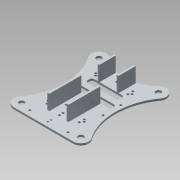
# Autodesk Inventor part: basebawahV2
Saved by Autodesk Inventor 2015 SP1 (Build 190203100, 203)
## iProperties
Created: 2015-01-14
Part Number: basebawahV2
Material: ABS Plastic
Document SubType Name: Modeling
Designer: Rafi Kurnia Putra
Density: 1.06 g/cm^3
Appearance: Default
Mass: 42.2508 g
Surface Area: 270.463 cm^2
Volume: 39.8593 cm^3
Author: Rafi Kurnia Putra
Autodesk Inventor part; units mm, degrees
ref_plane "YZ Plane" through (0, 0, 0) normal (1, 0, 0) x (0, 1, 0)
ref_plane "XZ Plane" through (0, 0, 0) normal (0, 1, 0) x (-1, 0, 0)
ref_plane "XY Plane" through (0, 0, 0) normal (0, 0, 1) x (1, 0, 0)
sketch "Sketch1" plane through (0, 0, 0) normal (0, 1, 0) x (-1, 0, 0)
  circle A0 centre (46.65, 60.8866) radius 4.25
  circle A1 centre (25.375, 42.175) radius 1.75
  circle A2 centre (28.625, 37.55) radius 1.75
  circle A3 centre (46.65, -60.8866) radius 4.25
  circle A4 centre (25.375, -42.175) radius 1.75
  circle A5 centre (28.625, -37.55) radius 1.75
  circle A6 centre (25.5, -34.24) radius 1.75
  circle A7 centre (25.5, 34.24) radius 1.75
  arc A8 (55.3297, 52.2069) -> (37.9702, 69.5664) centre (46.65, 60.8866) ccw
  arc A9 (37.9702, -69.5664) -> (55.3297, -52.2069) centre (46.65, -60.8866) ccw
  circle A10 centre (35.7091, 28.8987) radius 1.75
  circle A11 centre (38.6257, 37.55) radius 1.75
  circle A12 centre (28.8757, 53.55) radius 1.75
  line L0 (12.2659, 71.7451) -> (15.3224, 61.7249)
  arc A13 (22.1689, 58.6296) -> (37.9702, 69.5664) centre (0.0022, 107.5388) ccw
  arc A14 (15.3224, 61.7249) -> (22.1689, 58.6296) centre (20.1049, 63.1837) ccw
  circle A15 centre (-25.375, 42.175) radius 1.75
  circle A16 centre (-28.625, 37.55) radius 1.75
  circle A17 centre (-46.65, 60.8866) radius 4.25
  circle A18 centre (-25.375, -42.175) radius 1.75
  circle A19 centre (-28.625, -37.55) radius 1.75
  circle A20 centre (-46.65, -60.8866) radius 4.25
  circle A21 centre (-25.5, -34.24) radius 1.75
  circle A22 centre (-25.5, 34.24) radius 1.75
  arc A23 (-37.9702, 69.5664) -> (-55.3297, 52.2069) centre (-46.65, 60.8866) ccw
  arc A24 (-55.3297, -52.2069) -> (-37.9702, -69.5664) centre (-46.65, -60.8866) ccw
  circle A25 centre (-28.8757, 53.55) radius 1.75
  circle A26 centre (-38.6257, 37.55) radius 1.75
  circle A27 centre (-35.7091, 28.8987) radius 1.75
  line L1 (-12.2659, 71.7451) -> (-15.3224, 61.7249)
  arc A28 (-37.9702, 69.5664) -> (-22.1689, 58.6296) centre (-0.0022, 107.5388) ccw
  arc A29 (-22.1689, 58.6296) -> (-15.3224, 61.7249) centre (-20.1049, 63.1837) ccw
  circle A30 centre (0, 42.1912) radius 1.75
  arc A31 (37.9702, -69.5664) -> (-37.9702, -69.5664) centre (0, -107.5245) ccw
  line L2 (10.3529, 73.1616) -> (-10.3529, 73.1616)
  arc A32 (-55.3297, -52.2069) -> (-55.3297, 52.2069) centre (-134.1138, 0) ccw
  arc A33 (55.3297, 52.2069) -> (55.3297, -52.2069) centre (134.1138, 0) ccw
  arc A34 (12.2659, 71.7451) -> (10.3529, 73.1616) centre (10.3529, 71.1616) ccw
  arc A35 (-10.3529, 73.1616) -> (-12.2659, 71.7451) centre (-10.3529, 71.1616) ccw
  arc A36 (25.375, -21.8592) -> (21.875, -18.3592) centre (21.875, -21.8592) ccw
  arc A37 (21.875, -28.3427) -> (25.375, -24.8427) centre (21.875, -24.8427) ccw
  arc A38 (-25.375, -24.8427) -> (-21.875, -28.3427) centre (-21.875, -24.8427) ccw
  arc A39 (-21.875, -18.3592) -> (-25.375, -21.8592) centre (-21.875, -21.8592) ccw
  line L3 (-21.875, -18.3592) -> (21.875, -18.3592)
  line L4 (21.875, -28.3427) -> (-21.875, -28.3427)
  line L5 (-25.375, -21.8592) -> (-25.375, -24.8427)
  line L6 (25.375, -21.8592) -> (25.375, -24.8427)
  circle A40 centre (0, 61.1616) radius 1.25
  circle A41 centre (0, 66.1616) radius 1.25
  circle A42 centre (0, -42.1912) radius 1.75
  circle A43 centre (0, -48.0131) radius 1.75
  circle A44 centre (0, 48.0131) radius 1.75
  circle A45 centre (-34.6272, 13.8987) radius 1.75
  circle A46 centre (-34.6272, -13.8987) radius 1.75
  circle A47 centre (34.6272, 13.8987) radius 1.75
  circle A48 centre (34.6272, -13.8987) radius 1.75
  point P0 (57.609, 54.4281)
  point P1 (16.8957, 56.5674)
  point P2 (-0.0035, -53.835)
  point P3 (-57.609, 54.4281)
  point P4 (-16.8957, 56.5674)
  point P5 (0.0035, -53.835)
  point P6 (39.6019, 0)
  point P7 (-39.6019, 0)
  point P8 (25.25, -18.3592)
  point P9 (0, -18.3592)
  point P10 (-25.25, -18.3592)
  point P11 (46.65, -73.1616)
  point P12 (0, -73.1616)
  point P13 (46.65, 73.1616)
  point P14 (46.65, -73.1616)
  point P15 (-40.6295, 13.8987)
  dimension "d105" = 3.5
  dimension "d106" = 3.5
  dimension "d198" = 16
  dimension "d199" = 8.6513
  dimension "d244" = 5
  dimension "d247" = 79.2039
  dimension "d248" = 2
  dimension "d249" = 3.5
  dimension "d250" = 2.5
  dimension "d251" = 2.5
  dimension "d252" = 146.3233
  dimension "d253" = 146.3233
  dimension "d258" = 6.0022
  dimension "d259" = 27.7974
  dimension "d260" = 69.2545
  dimension "d263" = 5.8219
  dimension "d264" = 5.8219
  dimension "d265" = 5.8219
  dimension "d266" = 46.9879
  dimension "d267" = 12.0227
  dimension "d271" = 46.9879
  dimension "d272" = 12.0227
  constraints: 49 centre point, 42 point on circle, 14 end point, 6 tangent, 3 coincident, 2 equal radius, 2 point on line, 1 horizontal, 1 parallel, 1 perpendicular, 2 other
  measures "d105" diameter of A6
  measures "d106" diameter of A7
  measures "d198" vertical distance of A12.centre A11.centre
  measures "d199" vertical distance of A10.centre A11.centre
  measures "d244" radius of A14
  measures "d247" distance of point (-39.602, 0) point (39.602, 0)
  measures "d248" radius of A34
  measures "d249" radius of A36
  measures "d250" diameter of A40
  measures "d251" diameter of A41
  measures "d252" distance from line of L2 point (0, -73.162)
  measures "d253" distance of point (46.65, -73.162) point (46.65, 73.162)
  measures "d258" distance of A45.centre point (-40.629, 13.899)
  measures "d259" distance of A46.centre A45.centre
  measures "d260" distance of A47.centre A45.centre
  measures "d263" distance of A43.centre point (-0.004, -53.835)
  measures "d264" distance of A42.centre A43.centre
  measures "d265" distance of A30.centre A44.centre
  measures "d266" vertical distance of A45.centre A17.centre
  measures "d267" horizontal distance of A45.centre A17.centre
  measures "d271" vertical distance of A46.centre A20.centre
  measures "d272" horizontal distance of A46.centre A20.centre
extrude "Extrusion14" add sketch "Sketch1" along normal mid plane 3
sketch "Sketch14" plane through (0, -1.5, 0) normal (0, -1, 0) x (1, 0, 0)
  line L0 (31.815, 0) -> (31.815, -5.9519)
  arc A0 (28.315, -9.4519) -> (31.815, -5.9519) centre (28.315, -5.9519) ccw
  arc A1 (28.315, -9.4519) -> (28.625, -9.4382) centre (28.315, -5.9519) ccw
  line L1 (28.315, -9.4519) -> (0.0544, -9.4519)
  line L2 (28.315, 9.4519) -> (0.0544, 9.4519)
  arc A2 (31.815, 5.9519) -> (28.315, 9.4519) centre (28.315, 5.9519) ccw
  line L3 (31.815, 0) -> (31.815, 5.9519)
  arc A3 (28.625, 9.4382) -> (28.315, 9.4519) centre (28.315, 5.9519) ccw
  line L4 (-28.315, -9.4519) -> (-0.0544, -9.4519)
  line L5 (-31.815, 0) -> (-31.815, -5.9519)
  arc A4 (-31.815, -5.9519) -> (-28.315, -9.4519) centre (-28.315, -5.9519) ccw
  arc A5 (-28.625, -9.4382) -> (-28.315, -9.4519) centre (-28.315, -5.9519) ccw
  line L6 (-28.315, 9.4382) -> (-0.0544, 9.445)
  arc A6 (-28.315, 9.4382) -> (-28.6259, 9.4244) centre (-28.315, 5.9382) ccw
  arc A7 (-28.315, 9.4382) -> (-31.815, 5.9519) centre (-28.315, 5.9382) ccw
  line L7 (-31.815, 0) -> (-31.815, 5.9519)
  line L8 (-28.315, 9.4382) -> (28.625, 9.4382)
  line L9 (28.625, -9.4382) -> (-28.625, -9.4382)
  line L10 (-31.815, 5.9519) -> (-31.815, -5.9519)
  line L11 (31.815, 5.9519) -> (31.815, -5.9519)
  point P0 (0, 0)
  point P1 (0, 0)
  dimension "d268" = 63.63
  constraints: 24 end point, 20 point on circle, 8 centre point, 2 collinear, 2 parallel
  measures "d268" distance of L5.start L0.start
extrude "Extrusion15" cut sketch "Sketch14" against normal blind 3
sketch "Sketch15" plane through (0, 1.5, 0) normal (0, 1, 0) x (1, 0, 0)
  arc A0 (-46.65, -73.1616) -> (-37.9702, -69.5664) centre (-46.65, -60.8866) ccw
  arc A1 (-22.1689, -58.6296) -> (-37.9702, -69.5664) centre (-0.0022, -107.5388) ccw
  arc A2 (-15.3224, -61.7249) -> (-22.1689, -58.6296) centre (-20.1049, -63.1837) ccw
  line L0 (-15.3224, -61.7249) -> (-12.2659, -71.7451)
  arc A3 (-12.2659, -71.7451) -> (-10.3529, -73.1616) centre (-10.3529, -71.1616) ccw
  arc A4 (10.3529, -73.1616) -> (12.2659, -71.7451) centre (10.3529, -71.1616) ccw
  line L1 (12.2659, -71.7451) -> (15.3224, -61.7249)
  arc A5 (22.1689, -58.6296) -> (15.3224, -61.7249) centre (20.1049, -63.1837) ccw
  arc A6 (37.9702, -69.5664) -> (22.1689, -58.6296) centre (0.0022, -107.5388) ccw
  arc A7 (37.9702, -69.5664) -> (46.65, -73.1616) centre (46.65, -60.8866) ccw
  arc A8 (-46.65, -73.1616) -> (-37.9702, -69.5664) centre (-46.65, -60.8866) ccw
  line L2 (-46.65, -73.1616) -> (-10.3529, -73.1616)
  line L3 (10.3529, -73.1616) -> (46.65, -73.1616)
  line L4 (31.815, -5.9519) -> (31.815, 3.5)
  arc A9 (28.625, -9.4382) -> (31.815, -5.9519) centre (28.315, -5.9519) ccw
  line L5 (-28.315, -9.4382) -> (28.625, -9.4382)
  arc A10 (-31.815, -5.9519) -> (-28.315, -9.4382) centre (-28.315, -5.9382) ccw
  line L6 (-31.815, 3.5) -> (-31.815, -5.9519)
  line L7 (28.315, 0) -> (-28.315, 0)
  arc A11 (28.315, 0) -> (31.815, 3.5) centre (28.315, 3.5) ccw
  arc A12 (-31.815, 3.5) -> (-28.315, 0) centre (-28.315, 3.5) ccw
  dimension "d278" = 3.5
  dimension "d279" = 3.5
  constraints: 26 point on circle, 21 centre point, 16 end point, 4 tangent, 2 horizontal
  measures "d278" radius of A11
  measures "d279" radius of A12
extrude "Extrusion16" add sketch "Sketch15" against normal blind 3 contours A0 A1 A2 L0 A3 L2 | A4 L1 A5 A6 A7 L3
extrude "Extrusion17" add sketch "Sketch15" against normal blind 3 contours A9 L5 A10 L6 A12 L7 A11 L4
sketch "Sketch18" plane through (0, -1.5, 0) normal (0, -1, 0) x (1, 0, 0)
  arc A0 (23.8353, 3.8182) -> (25.559, 5.5419) centre (22.3772, 7) ccw projected
  line L0 (25.8772, 15.6487) -> (25.8772, 7) projected
  line L1 (22.3772, 3.5) -> (-22.3773, 3.5) projected
  circle A1 centre (20.8772, 8.5) radius 1.75
  circle A2 centre (-20.8772, 8.5) radius 1.75
  point P0 (0, 0)
  dimension "d285" = 5
  dimension "d286" = 5
  constraints: 2 centre point
  measures "d285" distance from line of A1.centre L1
  measures "d286" distance from line of A1.centre L0
extrude "Extrusion18" cut sketch "Sketch18" against normal up to next
sketch "Sketch19" plane through (0, -1.5, 0) normal (0, -1, 0) x (1, 0, 0)
  circle A0 centre (-30, 64.6618) radius 1.75
  line L0 (0, 0) -> (0, 78.7482)
  line L1 (-36.7454, 69.6618) -> (36.7451, 69.6619)
  circle A1 centre (-9, 28.5) radius 1.75
  line L2 (22.3772, 3.5) -> (-22.3773, 3.5)
  circle A2 centre (30, 64.6618) radius 1.75
  circle A3 centre (9, 28.5) radius 1.75
  dimension "d289" = 3.5
  dimension "d300" = 30
  dimension "d301" = 5
  dimension "d302" = 3.5
  dimension "d303" = 25
  dimension "d304" = 9
  constraints: 6 end point, 4 centre point, 2 symmetric about line, 1 vertical, 8 other
  measures "d289" diameter of A0
  measures "d300" distance from line of A0.centre L0
  measures "d301" distance from line of A0.centre L1
  measures "d302" diameter of A1
  measures "d303" distance from line of A1.centre L2
  measures "d304" distance from line of L0 A1.centre
sketch "Sketch20" plane through (0, -1.5, 0) normal (0, -1, 0) x (1, 0, 0)
  circle A0 centre (-35.7091, 28.8987) radius 1.75 projected
  circle A1 centre (-20.8772, 8.5) radius 1.75 projected
  circle A2 centre (20.8772, 8.5) radius 1.75 projected
  circle A3 centre (35.7091, 28.8987) radius 1.75 projected
  circle A4 centre (-38.6257, 37.55) radius 1.75 projected
  circle A5 centre (38.6257, 37.55) radius 1.75 projected
  circle A6 centre (-28.8757, 53.55) radius 1.75 projected
  circle A7 centre (28.8757, 53.55) radius 1.75 projected
  point P0 (0, 0)
extrude "Extrusion19" add sketch "Sketch20" against normal blind 3
extrude "Extrusion20" cut sketch "Sketch19" against normal through all
sketch "Sketch21" plane through (0, 1.5, 0) normal (0, 1, 0) x (1, 0, 0)
  line L0 (13.5, -50.3894) -> (13.5, 54.709)
  line L1 (-13.5, 54.0348) -> (-13.5, -50.3894)
  line L2 (16.5, -50.3894) -> (16.5, 55.1499)
  line L3 (-16.5, 55.1657) -> (-16.5, -50.3894)
  arc A0 (-16.5, 55.1657) -> (-13.5, 54.0348) centre (6.6191, 111.9486) ccw
  arc A1 (13.5, 54.709) -> (16.5, 55.1499) centre (6.6191, 111.9486) ccw
  line L4 (13.5, -50.3894) -> (16.5, -50.3894)
  line L5 (-16.5, -50.3894) -> (-13.5, -50.3894)
  point P0 (0, 0)
  dimension "d309" = 16.5
  dimension "d310" = 13.5
  dimension "d311" = 13.5
  dimension "d312" = 16.5
  constraints: 12 end point, 4 point on circle, 4 vertical, 2 centre point, 1 horizontal
  measures "d309" distance from line of point (0, 0) L2
  measures "d310" distance from line of point (0, 0) L0
  measures "d311" distance from line of point (0, 0) L1
  measures "d312" distance from line of L3 point (0, 0)
extrude "Extrusion23" add sketch "Sketch21" along normal blind 23.5
sketch "Sketch23" plane through (0, 1.5, 0) normal (0, -1, 0) x (1, 0, 0)
  line L0 (13.5, 0) -> (16.5, 0) projected
  line L1 (13.5, 0) -> (13.5, -9.4382) projected
  line L2 (13.5, -9.4382) -> (16.5, -9.4382) projected
  line L3 (16.5, -9.4382) -> (16.5, 0) projected
  line L4 (13.5, -28.3427) -> (16.5, -28.3427) projected
  line L5 (16.5, -28.3427) -> (16.5, -18.3592) projected
  line L6 (16.5, -18.3592) -> (13.5, -18.3592) projected
  line L7 (13.5, -18.3592) -> (13.5, -28.3427) projected
  line L8 (-16.5, 0) -> (-13.5, 0) projected
  line L9 (-16.5, -9.4382) -> (-16.5, 0) projected
  line L10 (-16.5, -9.4382) -> (-13.5, -9.4382) projected
  line L11 (-13.5, 0) -> (-13.5, -9.4382) projected
  line L12 (-16.5, -28.3427) -> (-13.5, -28.3427) projected
  line L13 (-13.5, -18.3592) -> (-13.5, -28.3427) projected
  line L14 (-13.5, -18.3592) -> (-16.5, -18.3592) projected
  line L15 (-16.5, -28.3427) -> (-16.5, -18.3592) projected
  point P0 (0, 0)
extrude "Extrusion24" cut sketch "Sketch23" against normal through all
sketch "Sketch24" plane through (0, 25, 0) normal (0, 1, 0) x (1, 0, 0)
  line L0 (-16.5, 9.4382) -> (-13.5, 9.4382) projected
  line L1 (-13.5, 9.4382) -> (-13.5, 18.3592) projected
  line L2 (-13.5, 18.3592) -> (-16.5, 18.3592) projected
  line L3 (-16.5, 18.3592) -> (-16.5, 9.4382) projected
  line L4 (16.5, 18.3592) -> (13.5, 18.3592) projected
  line L5 (13.5, 18.3592) -> (13.5, 9.4382) projected
  line L6 (13.5, 9.4382) -> (16.5, 9.4382) projected
  line L7 (16.5, 9.4382) -> (16.5, 18.3592) projected
  point P0 (0, 0)
extrude "Extrusion25" cut sketch "Sketch24" against normal blind 23.5
body "Solid10"
